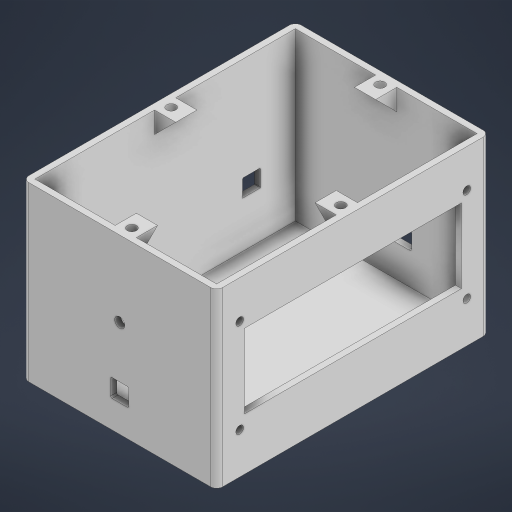
# Autodesk Inventor part: Case Bottom
Saved by Autodesk Inventor 2024 (Build 280153000, 153)
## iProperties
Created: 2023-06-21
Part Number: Case Bottom
Material: Generic
Document SubType Name: Modeling
Designer: Aryasetya
Density: 1 g/cm^3
Appearance: Default
Author: Aryasetya
Autodesk Inventor part; units mm, degrees
ref_plane "YZ Plane" through (0, 0, 0) normal (1, 0, 0) x (0, 1, 0)
ref_plane "XZ Plane" through (0, 0, 0) normal (0, 1, 0) x (-1, 0, 0)
ref_plane "XY Plane" through (0, 0, 0) normal (0, 0, 1) x (1, 0, 0)
sketch "Sketch1" plane through (0, 0, 0) normal (0, 1, 0) x (-1, 0, 0)
  line L0 (-30, -43) -> (30, -43)
  line L1 (30, -43) -> (30, 43)
  line L2 (30, 43) -> (-30, 43)
  line L3 (-30, 43) -> (-30, -43)
  line L4 (-30, -43) -> (30, 43) construction
  line L5 (30, -43) -> (-30, 43) construction
  line L6 (0, 43) -> (0, 45)
  line L7 (30, 0) -> (32, 0)
  line L8 (-30, -45) -> (30, -45)
  line L9 (32, -43) -> (32, 43)
  line L10 (30, 45) -> (-30, 45)
  line L11 (-32, 43) -> (-32, -43)
  line L12 (-32, -45) -> (32, 45) construction
  line L13 (32, -45) -> (-32, 45) construction
  arc A0 (-32, -43) -> (-30, -45) centre (-30, -43) ccw
  arc A1 (30, -45) -> (32, -43) centre (30, -43) ccw
  arc A2 (32, 43) -> (30, 45) centre (30, 43) ccw
  arc A3 (-30, 45) -> (-32, 43) centre (-30, 43) ccw
  point P0 (0, 0)
  dimension "d0" = 60
  dimension "d1" = 86
  dimension "d3" = 2
  dimension "d4" = 2
  dimension "d26" = 2
  constraints: 28 end point, 8 point on circle, 8 point on line, 8 tangent, 6 midpoint, 4 centre point, 4 parallel, 3 equal radius, 3 horizontal, 2 perpendicular, 1 vertical
  measures "d0" distance of L2.end L1.end
  measures "d1" distance of L1.end L0.end
  measures "d3" distance of L6.start L6.end
  measures "d4" distance of L7.start L7.end
  measures "d26" radius of A0
extrude "Extrusion1" add sketch "Sketch1" along normal blind 2
sketch "Sketch2" plane through (0, 2, 0) normal (0, 1, 0) x (1, 0, 0)
  line L0 (-30, -43) -> (30, -43)
  line L1 (30, -43) -> (30, 43)
  line L2 (30, 43) -> (-30, 43)
  line L3 (-30, 43) -> (-30, -43)
  line L4 (-30, -43) -> (30, 43) construction
  line L5 (30, -43) -> (-30, 43) construction
  line L6 (0, 43) -> (0, 45)
  line L7 (30, 0) -> (32, 0)
  line L8 (-30, -45) -> (30, -45)
  line L9 (32, -43) -> (32, 43)
  line L10 (30, 45) -> (-30, 45)
  line L11 (-32, 43) -> (-32, -43)
  line L12 (-32, -45) -> (32, 45) construction
  line L13 (32, -45) -> (-32, 45) construction
  arc A0 (32, 43) -> (30, 45) centre (30, 43) ccw
  arc A1 (-30, 45) -> (-32, 43) centre (-30, 43) ccw
  arc A2 (-32, -43) -> (-30, -45) centre (-30, -43) ccw
  arc A3 (30, -45) -> (32, -43) centre (30, -43) ccw
  point P0 (0, 0)
  point P1 (0, 0)
  dimension "d7" = 60
  dimension "d8" = 86
  dimension "d9" = 2
  dimension "d10" = 2
  dimension "d27" = 2
  constraints: 28 end point, 8 point on circle, 8 point on line, 8 tangent, 6 midpoint, 4 centre point, 4 parallel, 3 equal radius, 3 horizontal, 2 perpendicular, 1 vertical
  measures "d7" distance of L2.end L1.end
  measures "d8" distance of L1.end L0.end
  measures "d9" distance of L6.start L6.end
  measures "d10" distance of L7.start L7.end
  measures "d27" radius of A0
extrude "Extrusion2" add sketch "Sketch2" along normal blind 55 contours L0 L1 L7 L9 A3 L8 A2 L11 A1 L10 L6 L2 L3 | L1 L2 L6 L10 A0 L9 L7
sketch "Sketch3" plane through (32, 0, 45) normal (1, 0, 0) x (0, 0, -1)
  line L0 (2, 57) -> (88, 57) projected
  line L1 (2, 0) -> (88, 0) projected
  line L2 (107.729, 73.7861) -> (177.229, 73.7861)
  line L3 (106.879, 66.2861) -> (106.879, 57.2861)
  line L4 (106.879, 66.2861) -> (106.879, 72.9361)
  line L5 (106.879, 50.6361) -> (106.879, 57.2861)
  line L6 (177.229, 49.7861) -> (107.729, 49.7861)
  line L7 (178.079, 72.9361) -> (178.079, 50.6361)
  line L8 (142.479, 73.7861) -> (142.479, 49.7861)
  line L9 (178.079, 49.7861) -> (106.879, 49.7861)
  line L10 (106.879, 49.7861) -> (106.879, 73.7861)
  line L11 (106.879, 73.7861) -> (178.079, 73.7861)
  line L12 (178.079, 73.7861) -> (178.079, 49.7861)
  line L13 (178.079, 49.7861) -> (106.879, 73.7861) construction
  line L14 (106.879, 49.7861) -> (178.079, 73.7861) construction
  line L15 (177.069, 73.2861) -> (107.389, 73.2861)
  line L16 (82.6, 47) -> (52.1, 47)
  line L17 (7.6, 11) -> (82.6, 11)
  line L18 (7.6, 11) -> (82.6, 11)
  circle A0 centre (7.6, 44.5) radius 1.25
  line L19 (5.1, 44.5) -> (5.1, 13.5)
  line L20 (7.6, 11) -> (82.6, 11)
  line L21 (5.1, 11) -> (7.6, 11)
  circle A1 centre (7.6, 13.5) radius 1.25
  line L22 (5.1, 13.5) -> (5.1, 11)
  line L23 (82.6, 11) -> (85.1, 11)
  circle A2 centre (82.6, 13.5) radius 1.25
  circle A3 centre (82.6, 44.5) radius 1.25
  line L24 (85.1, 47) -> (82.6, 47)
  circle A4 centre (7.6, 44.5) radius 1.25
  line L25 (85.1, 47) -> (85.1, 11)
  line L26 (52.1, 47) -> (5.1, 47)
  line L27 (5.1, 47) -> (5.1, 44.5)
  line L28 (80.85, 17.25) -> (9.15, 17.25)
  line L29 (9.15, 17.25) -> (9.15, 41.75)
  line L30 (9.15, 41.75) -> (80.85, 41.75)
  line L31 (80.85, 41.75) -> (80.85, 17.25)
  line L32 (80.85, 17.25) -> (9.15, 41.75) construction
  line L33 (9.15, 17.25) -> (80.85, 41.75) construction
  point P0 (45, 0)
  point P1 (0, 57)
  point P2 (90, 57)
  point P3 (0, 0)
  point P4 (90, 0)
  point P5 (142.479, 61.7861)
  point P6 (45, 29.5)
  dimension "d21" = 71.7
  dimension "d22" = 24.5
  dimension "d100" = 2.5
  constraints: 64 end point, 7 midpoint, 5 centre point, 4 parallel, 3 horizontal, 3 perpendicular, 1 vertical
  measures "d21" distance of L29.end L30.end
  measures "d22" distance of L28.end L29.end
  measures "d100" diameter of A3
extrude "Extrusion3" cut sketch "Sketch3" against normal blind 10 contours A0 | A1 | A2 | A3 | L28 L29 L30 L31
sketch "Sketch4" plane through (32, 0, -45) normal (0, 0, -1) x (-1, 0, 0)
  line L0 (32, 0) -> (32, 12.5)
  line L1 (32, 12.5) -> (39.5, 12.5)
  line L2 (40.5, 13.5) -> (40.5, 17.5)
  line L3 (39.5, 18.5) -> (32, 18.5)
  line L4 (32, 18.5) -> (32, 12.5)
  line L5 (32, 12.5) -> (24.5, 12.5)
  line L6 (23.5, 13.5) -> (23.5, 17.5)
  line L7 (24.5, 18.5) -> (32, 18.5)
  arc A0 (24.5, 18.5) -> (23.5, 17.5) centre (24.5, 17.5) ccw
  arc A1 (23.5, 13.5) -> (24.5, 12.5) centre (24.5, 13.5) ccw
  arc A2 (39.5, 12.5) -> (40.5, 13.5) centre (39.5, 13.5) ccw
  arc A3 (40.5, 17.5) -> (39.5, 18.5) centre (39.5, 17.5) ccw
  point P0 (40.5, 18.5)
  point P1 (40.5, 12.5)
  point P2 (23.5, 18.5)
  point P3 (23.5, 12.5)
  dimension "d23" = 12.5
  dimension "d24" = 8.5
  dimension "d25" = 6
  dimension "d28" = 1
  constraints: 16 end point, 8 point on circle, 8 point on line, 8 tangent, 4 centre point, 3 equal radius, 2 parallel, 2 symmetric about line, 1 horizontal, 1 perpendicular, 1 vertical
  measures "d23" distance of L0.start L0.end
  measures "d24" distance of L3.end point (40.5, 18.5)
  measures "d25" distance of point (40.5, 18.5) point (40.5, 12.5)
  measures "d28" radius of A0
extrude "Extrusion4" cut sketch "Sketch4" against normal blind 10
sketch "Sketch5" plane through (-32, 0, -43) normal (-1, 0, 0) x (0, 0, 1)
  line L0 (0, 2) -> (86, 2) projected
  line L1 (86, 2) -> (66, 2)
  line L2 (66, 17) -> (72.05, 17)
  line L3 (66, 17) -> (59.95, 17)
  line L4 (58.95, 18) -> (58.95, 28)
  line L5 (59.95, 29) -> (72.05, 29)
  line L6 (73.05, 28) -> (73.05, 18)
  arc A0 (59.95, 29) -> (58.95, 28) centre (59.95, 28) ccw
  arc A1 (73.05, 28) -> (72.05, 29) centre (72.05, 28) ccw
  arc A2 (58.95, 18) -> (59.95, 17) centre (59.95, 18) ccw
  arc A3 (72.05, 17) -> (73.05, 18) centre (72.05, 18) ccw
  line L7 (66, 29) -> (66, 17)
  line L8 (66, 23) -> (58.95, 23)
  line L9 (78.85, 17.25) -> (7.15, 17.25) projected
  line L10 (66, 17) -> (67, 17) construction
  line L11 (15, 17) -> (16, 17)
  line L12 (17, 17) -> (12, 17)
  line L13 (11.5, 17.5) -> (11.5, 22.5)
  line L14 (12, 23) -> (17, 23)
  line L15 (17.5, 22.5) -> (17.5, 17.5)
  arc A4 (11.5, 17.5) -> (12, 17) centre (12, 17.5) ccw
  arc A5 (17, 17) -> (17.5, 17.5) centre (17, 17.5) ccw
  arc A6 (12, 23) -> (11.5, 22.5) centre (12, 22.5) ccw
  arc A7 (17.5, 22.5) -> (17, 23) centre (17, 22.5) ccw
  point P0 (43, 0)
  point P1 (73.05, 17)
  point P2 (58.95, 17)
  point P3 (58.95, 29)
  point P4 (14.5, 20)
  point P5 (17.5, 20)
  point P6 (11.5, 23)
  point P7 (11.5, 17)
  point P8 (17.5, 23)
  point P9 (11.567, 17.25)
  point P10 (17.433, 17.25)
  dimension "d31" = 20
  dimension "d32" = 15
  dimension "d33" = 7.05
  dimension "d34" = 12
  dimension "d35" = 1
  dimension "d83" = 50
  dimension "d89" = 6
  dimension "d90" = 6
  dimension "d91" = 0.5
  constraints: 28 end point, 16 point on circle, 16 tangent, 13 point on line, 8 centre point, 6 equal radius, 3 horizontal, 3 midpoint, 3 perpendicular, 2 parallel, 1 vertical
  measures "d31" distance of L0.end L1.end
  measures "d32" distance of L1.end L2.start
  measures "d33" distance of L2.start point (73.05, 17)
  measures "d34" distance of point (58.95, 17) point (58.95, 29)
  measures "d35" radius of A0
  measures "d83" distance of L2.start L11.end
  measures "d89" distance of point (11.5, 23) point (17.5, 23)
  measures "d90" distance of point (11.5, 17) point (11.5, 23)
  measures "d91" radius of A4
extrude "Extrusion5" cut sketch "Sketch5" against normal blind 10 contours L7 L9 A3 L2 | L9 A4 L13 A6 L14 A7 L15 A5 | L3 A2 L9 L7 | L9 A2 L4 L8 L7 | L7 L5 A1 L6 A3 L9 | L8 L4 A0 L5 L7
sketch "Sketch6" plane through (-30, 2, 43) normal (1, 0, 0) x (0, 0, -1)
  line L0 (0, 55) -> (86, 55) projected
  line L1 (43, 55) -> (43, 48)
  line L2 (43, 48) -> (39.5, 48)
  line L3 (39.5, 48) -> (39.5, 55)
  line L4 (43, 48) -> (46.5, 48)
  line L5 (46.5, 48) -> (46.5, 55)
  point P0 (43, -2)
  dimension "d38" = 7
  dimension "d39" = 3.5
  constraints: 10 end point, 2 symmetric about line, 1 horizontal, 1 midpoint, 1 perpendicular, 1 point on line, 1 vertical
  measures "d38" distance of L1.start L1.end
  measures "d39" distance of L1.end L2.end
extrude "Extrusion6" add sketch "Sketch6" along normal blind 7
sketch "Sketch8" plane through (-30, 50, 3.5) normal (0, 0, 1) x (1, 0, 0)
  line L0 (7, 7) -> (7, 0) projected
  line L1 (0, 0) -> (7, 0) projected
  line L2 (0, 0) -> (0, 7) projected
  line L3 (0, 7) -> (7, 7) projected
  line L4 (7, 7) -> (0, 0)
  point P0 (30, -50)
  constraints: 2 end point
extrude "Extrusion7" cut sketch "Sketch8" against normal blind 7 contours L0 L1 L4
sketch "Sketch9" plane through (0, 57, 0) normal (0, 1, 0) x (1, 0, 0)
  line L0 (-30, 3.5) -> (-23, 3.5) projected
  line L1 (-30, -3.5) -> (-23, -3.5) projected
  line L2 (-23, 3.5) -> (-23, -3.5) projected
  line L3 (-30, 3.5) -> (-30, -3.5)
  line L4 (-30, 43) -> (-30, -43) projected
  line L5 (-23, 0) -> (-28, 0)
  circle A0 centre (-28, 0) radius 1.5
  point P0 (0, 0)
  dimension "d47" = 5
  dimension "d48" = 3
  constraints: 4 end point, 1 centre point, 1 coincident, 1 collinear, 1 horizontal, 1 midpoint
  measures "d47" distance of L5.start L5.end
  measures "d48" diameter of A0
extrude "Extrusion8" cut sketch "Sketch9" against normal blind 3 contours A0
sketch "Sketch11" plane through (-30, 2, -43) normal (0, 0, 1) x (1, 0, 0)
  line L0 (0, 55) -> (60, 55) projected
  line L1 (30, 55) -> (30, 48)
  line L2 (30, 48) -> (33.5, 48)
  line L3 (33.5, 48) -> (33.5, 55)
  line L4 (30, 48) -> (26.5, 48)
  line L5 (26.5, 48) -> (26.5, 55)
  point P0 (30, -2)
  dimension "d49" = 7
  dimension "d50" = 3.5
  dimension "d51" = 3.5
  constraints: 10 end point, 3 perpendicular, 2 point on line, 1 horizontal, 1 midpoint, 1 vertical
  measures "d49" distance of L1.start L1.end
  measures "d50" distance of L1.end L2.end
  measures "d51" distance of L1.end L4.end
extrude "Extrusion9" add sketch "Sketch11" along normal blind 7
sketch "Sketch12" plane through (-3.5, 50, -43) normal (-1, 0, 0) x (0, 0, 1)
  line L0 (7, 7) -> (7, 0) projected
  line L1 (0, 0) -> (7, 0) projected
  line L2 (7, 7) -> (0, 0)
  point P0 (43, -50)
  constraints: 2 end point
extrude "Extrusion10" cut sketch "Sketch12" against normal blind 7
sketch "Sketch13" plane through (0, 57, 0) normal (0, 1, 0) x (1, 0, 0)
  line L0 (3.5, 36) -> (-3.5, 36) projected
  line L1 (0, 36) -> (0, 41)
  circle A0 centre (0, 41) radius 1.5
  point P0 (0, 0)
  dimension "d56" = 5
  dimension "d57" = 3
  constraints: 2 end point, 1 centre point, 1 coincident, 1 midpoint, 1 vertical
  measures "d56" distance of L1.start L1.end
  measures "d57" diameter of A0
extrude "Extrusion11" cut sketch "Sketch13" against normal blind 3
sketch "Sketch14" plane through (30, 2, -43) normal (-1, 0, 0) x (0, 0, 1)
  line L0 (0, 55) -> (86, 55) projected
  line L1 (43, 55) -> (43, 48)
  line L2 (43, 48) -> (46.5, 48)
  line L3 (46.5, 48) -> (46.5, 55)
  line L4 (43, 48) -> (39.5, 48)
  line L5 (39.5, 48) -> (39.5, 55)
  point P0 (43, -2)
  dimension "d60" = 7
  dimension "d61" = 3.5
  constraints: 10 end point, 2 perpendicular, 2 symmetric about line, 1 midpoint, 1 point on line, 1 vertical
  measures "d60" distance of L1.start L1.end
  measures "d61" distance of L1.end L2.end
extrude "Extrusion12" add sketch "Sketch14" along normal blind 7
sketch "Sketch17" plane through (30, 50, -3.5) normal (0, 0, -1) x (-1, 0, 0)
  line L0 (7, 7) -> (7, 0) projected
  line L1 (0, 0) -> (7, 0) projected
  line L2 (0, 0) -> (7, 7)
  point P0 (30, -50)
  constraints: 2 end point
extrude "Extrusion13" cut sketch "Sketch17" against normal blind 7
sketch "Sketch18" plane through (0, 57, 0) normal (0, 1, 0) x (1, 0, 0)
  line L0 (23, -3.5) -> (23, 3.5) projected
  line L1 (23, 0) -> (28, 0)
  circle A0 centre (28, 0) radius 1.5
  point P0 (0, 0)
  dimension "d66" = 5
  dimension "d67" = 3
  constraints: 2 end point, 1 centre point, 1 coincident, 1 horizontal, 1 midpoint
  measures "d66" distance of L1.start L1.end
  measures "d67" diameter of A0
extrude "Extrusion14" cut sketch "Sketch18" against normal blind 3
sketch "Sketch19" plane through (30, 2, 43) normal (0, 0, -1) x (-1, 0, 0)
  line L0 (0, 55) -> (60, 55) projected
  line L1 (30, 55) -> (30, 48)
  line L2 (30, 48) -> (33.5, 48)
  line L3 (33.5, 48) -> (33.5, 55)
  line L4 (30, 48) -> (26.5, 48)
  line L5 (26.5, 48) -> (26.5, 55)
  point P0 (30, -2)
  dimension "d70" = 7
  dimension "d71" = 3.5
  constraints: 10 end point, 2 perpendicular, 2 symmetric about line, 1 midpoint, 1 point on line, 1 vertical
  measures "d70" distance of L1.start L1.end
  measures "d71" distance of L1.end L2.end
extrude "Extrusion15" add sketch "Sketch19" along normal blind 7
sketch "Sketch20" plane through (3.5, 50, 43) normal (1, 0, 0) x (0, 0, -1)
  line L0 (7, 7) -> (7, 0) projected
  line L1 (0, 0) -> (7, 0) projected
  line L2 (0, 0) -> (7, 7)
  point P0 (43, -50)
  constraints: 2 end point
extrude "Extrusion16" cut sketch "Sketch20" against normal blind 7
sketch "Sketch21" plane through (0, 57, 0) normal (0, 1, 0) x (1, 0, 0)
  line L0 (-3.5, -36) -> (3.5, -36) projected
  line L1 (-3.5, -43) -> (-3.5, -36) projected
  line L2 (3.5, -43) -> (3.5, -36) projected
  line L3 (0, -36) -> (0, -41)
  circle A0 centre (0, -41) radius 1.5
  point P0 (0, 0)
  dimension "d76" = 5
  dimension "d77" = 3
  constraints: 2 end point, 1 centre point, 1 coincident, 1 midpoint, 1 vertical
  measures "d76" distance of L3.start L3.end
  measures "d77" diameter of A0
extrude "Extrusion17" cut sketch "Sketch21" against normal blind 3
sketch "Sketch23" plane through (-30, 0, 45) normal (0, 0, 1) x (1, 0, 0)
  line L0 (0, 2) -> (60, 2) projected
  line L1 (0, 57) -> (60, 57) projected
  line L2 (30, 2) -> (30, 12)
  circle A0 centre (30, 32) radius 1.65
  line L3 (32.5, 9) -> (27.5, 9)
  line L4 (27, 9.5) -> (27, 14.5)
  line L5 (27.5, 15) -> (32.5, 15)
  line L6 (33, 14.5) -> (33, 9.5)
  line L7 (33, 9) -> (27, 15) construction
  line L8 (27, 9) -> (33, 15) construction
  arc A1 (33, 14.5) -> (32.5, 15) centre (32.5, 14.5) ccw
  arc A2 (27.5, 15) -> (27, 14.5) centre (27.5, 14.5) ccw
  arc A3 (27, 9.5) -> (27.5, 9) centre (27.5, 9.5) ccw
  arc A4 (32.5, 9) -> (33, 9.5) centre (32.5, 9.5) ccw
  point P0 (30, 0)
  dimension "d92" = 10
  dimension "d94" = 3.3
  dimension "d95" = 6
  dimension "d96" = 6
  dimension "d97" = 0.5
  constraints: 14 end point, 8 point on circle, 8 point on line, 8 tangent, 5 centre point, 3 equal radius, 3 midpoint, 2 parallel, 1 horizontal, 1 perpendicular
  measures "d92" distance of L2.start L2.end
  measures "d94" diameter of A0
  measures "d95" distance of L7.end L8.end
  measures "d96" distance of L8.start L7.end
  measures "d97" radius of A1
extrude "Extrusion18" cut sketch "Sketch23" against normal blind 10
body "Solid1"
